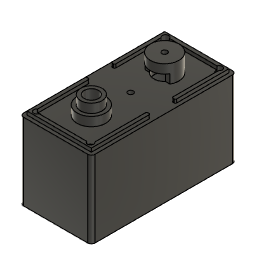
MG996R_Shell_Middle v8 (Autodesk Fusion 360 design; units mm, degrees)
Autodesk Fusion 360 part; units mm, degrees
sketch "Sketch1" plane through (0, 0, 0) normal (0, 0, 1) x (1, 0, 0)
  line L0 (10, 20.25) -> (-10, 20.25)
  line L1 (-10, 20.25) -> (-10, -20.25)
  line L2 (-10, -20.25) -> (10, -20.25)
  line L3 (10, -20.25) -> (10, 20.25)
  line L4 (10, 20.25) -> (-10, -20.25) construction
  line L5 (-10, 20.25) -> (10, -20.25) construction
  dimension "d1" = 20
  dimension "d2" = 40.5
  constraint horizontal L0
  constraint perpendicular L0 L1
  constraint parallel L0 L2
  constraint parallel L1 L3
  constraint coincident L4 origin
  constraint coincident L5 origin
  measures "d1" distance of L0.start L0.end
  measures "d2" distance of L0.end L1.end
extrude "Extrude1" add sketch "Sketch1" along normal blind 21.5
sketch "Sketch2" plane through (0, 0, 21.5) normal (0, 0, 1) x (-1, 0, 0)
  line L0 (-10, 20.25) -> (-10, -20.25)
  line L1 (-10, -20.25) -> (10, -20.25)
  line L2 (10, -20.25) -> (10, 20.25)
  line L3 (10, 20.25) -> (-10, 20.25)
  line L4 (-8, -18.25) -> (8, -18.25)
  line L5 (8, -18.25) -> (8, 18.25)
  line L6 (8, 18.25) -> (-8, 18.25)
  line L7 (-8, 18.25) -> (-8, -18.25)
  line L8 (-8, -18.25) -> (8, 18.25) construction
  line L9 (8, -18.25) -> (-8, 18.25) construction
  line L10 (-9, -19.25) -> (9, -19.25)
  line L11 (9, -19.25) -> (9, 19.25)
  line L12 (9, 19.25) -> (-9, 19.25)
  line L13 (-9, 19.25) -> (-9, -19.25)
  line L14 (-9, -19.25) -> (9, 19.25) construction
  line L15 (9, -19.25) -> (-9, 19.25) construction
  dimension "d5" = 1
  dimension "d6" = 1
  dimension "d7" = 1
  dimension "d8" = 1
  constraint horizontal L4
  constraint perpendicular L4 L5
  constraint parallel L4 L6
  constraint parallel L5 L7
  constraint coincident L8 origin
  constraint coincident L9 origin
  constraint horizontal L10
  constraint perpendicular L10 L11
  constraint parallel L10 L12
  constraint parallel L11 L13
  constraint coincident L14 origin
  constraint coincident L15 origin
  measures "d5" distance of L4 L10
  measures "d6" distance of L7 L13
  measures "d7" distance of L0 L13
  measures "d8" distance of L1 L10
extrude "Extrude2" add sketch "Sketch2" along normal blind 1 contours L10 L11 L12 L13
sketch "Sketch3" plane through (0, 0, 21.5) normal (0, 0, 1) x (-1, 0, 0)
  line L0 (-8, -18.25) -> (8, -18.25)
  line L1 (8, -18.25) -> (8, 18.25)
  line L2 (8, 18.25) -> (-8, 18.25)
  line L3 (-8, 18.25) -> (-8, -18.25)
  circle A0 centre (0, 10.25) radius 2
  line L4 (10, 20.25) -> (-10, 20.25)
  circle A1 centre (0, -0.75) radius 0.75
  circle A2 centre (0, -10.25) radius 3
  line L5 (-10, -20.25) -> (10, -20.25)
  circle A3 centre (0, -10.25) radius 4
  circle A4 centre (0, 10.25) radius 4
  dimension "d11" = 4
  dimension "d12" = 10
  dimension "d13" = 11
  dimension "d14" = 9.5
  dimension "d16" = 10
  dimension "d17" = 1.5
  dimension "d18" = 6
  dimension "d19" = 8
  dimension "d20" = 8
  constraint vertical A1.centre A2.centre
  constraint vertical A0.centre A1.centre
  constraint vertical origin A1.centre
  constraint concentric A2 A3
  constraint concentric A0 A4
  measures "d11" diameter of A0
  measures "d12" distance of A0.centre L4
  measures "d13" vertical distance of A0.centre A1.centre
  measures "d14" distance of A1.centre A2.centre
  measures "d16" distance of A2.centre L5
  measures "d17" diameter of A1
  measures "d18" diameter of A2
  measures "d19" diameter of A4
  measures "d20" diameter of A3
extrude "Extrude3" add sketch "Sketch3" along normal blind 5 contours A3
extrude "Extrude4" add sketch "Sketch3" along normal blind 5 contours A4
sketch "Sketch4" plane through (0, 0, 26.5) normal (0, 0, 1) x (-1, 0, 0)
  circle A0 centre (0, 10.25) radius 2
  circle A1 centre (0, 10.25) radius 4
  circle A2 centre (0, 10.25) radius 3
  dimension "d25" = 6
  constraint concentric A0 A2
  measures "d25" diameter of A2
extrude "Extrude5" cut sketch "Sketch4" against normal blind 2.5 contours A1
extrude "Extrude6" cut sketch "Sketch3" against normal blind 1.5 contours A1
sketch "Sketch5" plane through (0, 0, 0) normal (0, 0, -1) x (1, 0, 0)
  line L0 (10, -20.25) -> (10, 20.25)
  line L1 (10, 20.25) -> (-10, 20.25)
  line L2 (-10, 20.25) -> (-10, -20.25)
  line L3 (-10, -20.25) -> (10, -20.25)
  line L4 (7.5, 18) -> (-7.5, 18) construction
  line L5 (-7.5, 18) -> (-7.5, -18) construction
  line L6 (-7.5, -18) -> (7.5, -18) construction
  line L7 (7.5, -18) -> (7.5, 18) construction
  line L8 (7.5, 18) -> (-7.5, -18) construction
  line L9 (-7.5, 18) -> (7.5, -18) construction
  circle A0 centre (-7.5, 18) radius 0.875
  circle A1 centre (7.5, 18) radius 0.875
  circle A2 centre (7.5, -18) radius 0.875
  circle A3 centre (-7.5, -18) radius 0.875
  dimension "d30" = 15
  dimension "d31" = 36
  dimension "d32" = 1.75
  constraint horizontal L4
  constraint perpendicular L4 L5
  constraint parallel L4 L6
  constraint parallel L5 L7
  constraint coincident L8 origin
  constraint coincident L9 origin
  constraint coincident L4.end L5.start
  constraint coincident L4.start L7.end
  constraint coincident L6.end L7.start
  constraint coincident L5.end L6.start
  constraint equal A0 A1
  constraint equal A1 A2
  constraint equal A2 A3
  measures "d30" distance of L4.start L4.end
  measures "d31" distance of L4.end L5.end
  measures "d32" diameter of A3
extrude "Extrude7" cut sketch "Sketch5" against normal blind 27 contours A0 | A1 | A2 | A3
sketch "Sketch6" plane through (0, 0, 0) normal (0, 0, -1) x (1, 0, 0)
  circle A0 centre (7.5, 18) radius 0.875
  circle A1 centre (7.5, -18) radius 0.875
  circle A2 centre (-7.5, 18) radius 0.875
  circle A3 centre (-7.5, -18) radius 0.875
  line L0 (10, -20.25) -> (10, 20.25)
  line L1 (10, 20.25) -> (-10, 20.25)
  line L2 (-10, 20.25) -> (-10, -20.25)
  line L3 (-10, -20.25) -> (10, -20.25)
  circle A4 centre (-7.5, 18) radius 1.875
  circle A5 centre (7.5, 18) radius 1.875
  circle A6 centre (7.5, -18) radius 1.875
  circle A7 centre (-7.5, -18) radius 1.875
  line L4 (9, 19.25) -> (-9, 19.25)
  line L5 (-9, 19.25) -> (-9, -19.25)
  line L6 (-9, -19.25) -> (9, -19.25)
  line L7 (9, -19.25) -> (9, 19.25)
  line L8 (9, 19.25) -> (-9, -19.25) construction
  line L9 (-9, 19.25) -> (9, -19.25) construction
  dimension "d35" = 3.75
  dimension "d36" = 1
  dimension "d37" = 1
  constraint concentric A2 A4
  constraint concentric A0 A5
  constraint concentric A1 A6
  constraint concentric A3 A7
  constraint equal A4 A7
  constraint equal A4 A5
  constraint equal A5 A6
  constraint horizontal L4
  constraint perpendicular L4 L5
  constraint parallel L4 L6
  constraint parallel L5 L7
  constraint coincident L8 origin
  constraint coincident L9 origin
  measures "d35" diameter of A7
  measures "d36" distance of L1 L4
  measures "d37" distance of L2 L5
extrude "Extrude8" cut sketch "Sketch6" against normal up to surface (19.5 mm away) contours A4 A5 A6 A7 L4 L5 L6 L7
extrude "Extrude9" cut 1 faces at (0.1483, -10.9, 21.5) along direction (0, 0, -1) blind 15
sketch "Sketch8" plane through (0, 0, 26.5) normal (0, 0, 1) x (-1, 0, 0)
  circle A0 centre (0, -10.25) radius 3
  circle A1 centre (0, -10.25) radius 4
  circle A2 centre (0, -10.25) radius 4
  constraint concentric A0 A2
extrude "Extrude10" add sketch "Sketch8" against normal blind 2.5 contours A0
ref_plane "WorkPlane1" through (0, 6.25, 22) normal (0, -1, 0) x (1, 0, 0)
sketch "Sketch10" plane through (0, 6.25, 22) normal (0, -1, 0) x (1, 0, 0)
  line L0 (-4, 2) -> (4, 2)
  line L1 (4, 2) -> (4, -0.5)
  line L2 (4, -0.5) -> (-4, -0.5)
  line L3 (-4, -0.5) -> (-4, 2)
  constraint horizontal L0
  constraint vertical L1
  constraint horizontal L2
  constraint vertical L3
extrude "Extrude11" cut sketch "Sketch10" against normal blind 2
sketch "Sketch11" plane through (0, 0, 26.5) normal (0, 0, 1) x (-1, 0, 0)
  circle A0 centre (0, -10.25) radius 4
  circle A1 centre (0, -10.25) radius 0.75
  dimension "d47" = 1.5
  constraint concentric A0 A1
  measures "d47" diameter of A1
extrude "Extrude12" cut sketch "Sketch11" against normal blind 1.5 contours A1
sketch "Sketch12" plane through (0, 0, 21.5) normal (0, 0, 1) x (-1, 0, 0)
  arc A0 (-3.4641, -8.25) -> (3.4641, -8.25) centre (0, -10.25) ccw
  line L0 (-3.4641, -8.25) -> (-2.2361, -8.25)
  arc A1 (-2.2361, -8.25) -> (2.2361, -8.25) centre (0, -10.25) ccw
  line L1 (2.2361, -8.25) -> (3.4641, -8.25)
  arc A2 (-8, 17.2819) -> (-6.6615, 18.25) centre (-7.5, 18) ccw
  line L2 (-8, 17.2819) -> (-8, -17.2819)
  arc A3 (-6.6615, -18.25) -> (-8, -17.2819) centre (-7.5, -18) ccw
  line L3 (-6.6615, -18.25) -> (6.6615, -18.25)
  arc A4 (8, -17.2819) -> (6.6615, -18.25) centre (7.5, -18) ccw
  line L4 (8, -17.2819) -> (8, 17.2819)
  arc A5 (6.6615, 18.25) -> (8, 17.2819) centre (7.5, 18) ccw
  line L5 (6.6615, 18.25) -> (-6.6615, 18.25)
  circle A6 centre (0, -0.75) radius 0.75
  circle A7 centre (0, 10.25) radius 4
  circle A8 centre (0, -10.25) radius 3
  dimension "d50" = 6
  constraint concentric A0 A8
  measures "d50" diameter of A8
extrude "Extrude13" cut sketch "Sketch12" against normal blind 4 contours A1 A8
sketch "Sketch13" plane through (0, 0, 21.5) normal (0, 0, 1) x (-1, 0, 0)
  arc A0 (2.2361, -8.25) -> (-2.2361, -8.25) centre (0, -10.25) ccw
  line L0 (2.2361, -8.25) -> (3.4641, -8.25)
  arc A1 (-3.4641, -8.25) -> (3.4641, -8.25) centre (0, -10.25) ccw
  line L1 (-3.4641, -8.25) -> (-2.2361, -8.25)
  arc A2 (-8, 17.2819) -> (-6.6615, 18.25) centre (-7.5, 18) ccw
  line L2 (-8, 17.2819) -> (-8, -17.2819)
  arc A3 (-6.6615, -18.25) -> (-8, -17.2819) centre (-7.5, -18) ccw
  line L3 (-6.6615, -18.25) -> (6.6615, -18.25)
  arc A4 (8, -17.2819) -> (6.6615, -18.25) centre (7.5, -18) ccw
  line L4 (8, -17.2819) -> (8, 17.2819)
  arc A5 (6.6615, 18.25) -> (8, 17.2819) centre (7.5, 18) ccw
  line L5 (6.6615, 18.25) -> (-6.6615, 18.25)
  circle A6 centre (0, -0.75) radius 0.75
  circle A7 centre (0, 10.25) radius 4
  line L6 (-12.9231, -4.25) -> (12.9231, -4.25)
  line L7 (12.9231, -4.25) -> (12.9231, 2.75)
  line L8 (12.9231, 2.75) -> (-12.9231, 2.75)
  line L9 (-12.9231, 2.75) -> (-12.9231, -4.25)
  line L10 (-12.9231, -4.25) -> (12.9231, 2.75) construction
  line L11 (12.9231, -4.25) -> (-12.9231, 2.75) construction
  point P0 (0, -0.75)
  dimension "d53" = 7
  constraint horizontal L6
  constraint perpendicular L6 L7
  constraint parallel L6 L8
  constraint parallel L7 L9
  constraint coincident L10 P0
  constraint coincident L11 P0
  constraint coincident P0 A6.centre
  measures "d53" distance of L6.end L7.end
extrude "Extrude14" cut sketch "Sketch13" along normal blind 3 contours L2 L6 L8 L9 | L4 L6 L7 L8
fillet "Fillet1" radius 0.35 8 edges at (-9, 4.25, 22) (-8, 4.25, 22) (-9, -2.75, 22) (-8, -2.75, 22) (8, 4.25, 22) (9, 4.25, 22) (8, -2.75, 22) (9, -2.75, 22)
fillet "Fillet2" radius 1 4 edges at (-10, -20.25, 10.75) (10, -20.25, 10.75) (-10, 20.25, 10.75) (10, 20.25, 10.75)
sketch "Sketch14" plane through (0, 0, 19.5) normal (0, 0, -1) x (1, 0, 0)
  circle A0 centre (0, -10.25) radius 3
  circle A1 centre (0, 10.25) radius 2
  arc A2 (-6.1025, -19.25) -> (-9, -16.875) centre (-7.5, -18) ccw
  line L0 (-6.1025, -19.25) -> (6.1025, -19.25)
  arc A3 (9, -16.875) -> (6.1025, -19.25) centre (7.5, -18) ccw
  line L1 (9, -16.875) -> (9, 16.875)
  arc A4 (6.1025, 19.25) -> (9, 16.875) centre (7.5, 18) ccw
  line L2 (6.1025, 19.25) -> (-6.1025, 19.25)
  arc A5 (-9, 16.875) -> (-6.1025, 19.25) centre (-7.5, 18) ccw
  line L3 (-9, 16.875) -> (-9, -16.875)
  circle A6 centre (0, -10.25) radius 8.5
  circle A7 centre (0, -10.25) radius 9.5
  dimension "d60" = 17
  dimension "d61" = 1
  constraint concentric A0 A6
  constraint concentric A6 A7
  measures "d60" diameter of A6
  measures "d61" distance of A6 A7
extrude "Extrude15" add sketch "Sketch14" along normal blind 12 contours A2 L0 A3 L1 L3 A7
sketch "Sketch15" plane through (0, 0, 19.5) normal (0, 0, -1) x (1, 0, 0)
  circle A0 centre (0, 10.25) radius 2
  arc A1 (9, -7.2086) -> (-9, -7.2086) centre (0, -10.25) ccw
  line L0 (9, -7.2086) -> (9, 16.875)
  arc A2 (6.1025, 19.25) -> (9, 16.875) centre (7.5, 18) ccw
  line L1 (6.1025, 19.25) -> (-6.1025, 19.25)
  arc A3 (-9, 16.875) -> (-6.1025, 19.25) centre (-7.5, 18) ccw
  line L2 (-9, 16.875) -> (-9, -7.2086)
  line L3 (5, 15.75) -> (-5, 15.75)
  line L4 (-5, 15.75) -> (-5, 4.75)
  line L5 (-5, 4.75) -> (5, 4.75)
  line L6 (5, 4.75) -> (5, 15.75)
  line L7 (5, 15.75) -> (-5, 4.75) construction
  line L8 (-5, 15.75) -> (5, 4.75) construction
  line L9 (6, 16.75) -> (-6, 16.75)
  line L10 (-6, 16.75) -> (-6, 3.75)
  line L11 (-6, 3.75) -> (6, 3.75)
  line L12 (6, 3.75) -> (6, 16.75)
  line L13 (6, 16.75) -> (-6, 3.75) construction
  line L14 (-6, 16.75) -> (6, 3.75) construction
  point P0 (0, 10.25)
  point P1 (0, 10.25)
  dimension "d64" = 10
  dimension "d65" = 11
  dimension "d66" = 1
  dimension "d67" = 1
  constraint horizontal L3
  constraint perpendicular L3 L4
  constraint parallel L3 L5
  constraint parallel L4 L6
  constraint coincident L7 P1
  constraint coincident L8 P1
  constraint coincident P0 A0.centre
  constraint horizontal L9
  constraint perpendicular L9 L10
  constraint parallel L9 L11
  constraint parallel L10 L12
  constraint coincident L13 P1
  constraint coincident L14 P1
  constraint coincident P1 P0
  measures "d64" distance of L3.start L3.end
  measures "d65" distance of L3.start L5.end
  measures "d66" distance of L6 L12
  measures "d67" distance of L3 L9
extrude "Extrude16" add sketch "Sketch15" along normal blind 5 contours L9 L10 L11 L12
equation "d35 = 1.75 mm + 2 mm"
